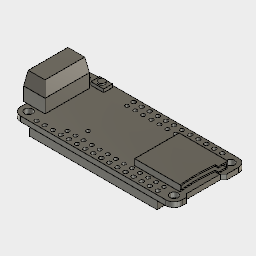
3436 Adafruit Music Maker Amp Feather Wing (Autodesk Fusion 360 design; units mm, degrees)
Autodesk Fusion 360 part; units mm, degrees
sketch "Adafruit VS1053 Amp FeatherWing" plane through (0, 0, 0) normal (0, 0, 1) x (1, 0, 0)
  line L0 (50.8, 16.637) -> (49.784, 15.621)
  line L1 (50.8, 3.937) -> (50.8, 2.54)
  line L2 (48.26, 0) -> (2.54, 0)
  line L3 (49.784, 15.621) -> (49.784, 4.953)
  line L4 (49.784, 4.953) -> (50.8, 3.937)
  line L5 (50.8, 20.32) -> (50.8, 16.637)
  circle A0 centre (48.26, 20.32) radius 1.27
  arc A1 (48.26, 0) -> (50.8, 2.54) centre (48.26, 2.54) ccw
  line L6 (2.54, 22.86) -> (48.26, 22.86)
  arc A2 (50.8, 20.32) -> (48.26, 22.86) centre (48.26, 20.32) ccw
  line L7 (0, 2.54) -> (0, 20.32)
  arc A3 (2.54, 22.86) -> (0, 20.32) centre (2.54, 20.32) ccw
  circle A4 centre (48.26, 2.54) radius 1.27
  arc A5 (0, 2.54) -> (2.54, 0) centre (2.54, 2.54) ccw
  circle A6 centre (13.97, 3.302) radius 0.8382
  circle A7 centre (16.51, 3.302) radius 0.8382
  circle A8 centre (19.05, 3.302) radius 0.8382
  circle A9 centre (39.37, 1.27) radius 0.889
  circle A10 centre (21.59, 3.302) radius 0.8382
  circle A11 centre (16.51, 3.302) radius 0.8382
  circle A12 centre (13.97, 3.302) radius 0.8382
  circle A13 centre (17.272, 6.5405) radius 0.8382
  circle A14 centre (19.05, 3.302) radius 0.8382
  circle A15 centre (2.159, 9.701) radius 1.0922
  circle A16 centre (29.21, 1.27) radius 0.889
  circle A17 centre (29.21, 1.27) radius 0.889
  circle A18 centre (44.45, 1.27) radius 0.889
  circle A19 centre (44.45, 1.27) radius 0.889
  circle A20 centre (26.67, 1.27) radius 0.889
  circle A21 centre (34.29, 21.59) radius 0.889
  circle A22 centre (34.29, 21.59) radius 0.889
  circle A23 centre (24.13, 3.302) radius 0.8382
  circle A24 centre (36.83, 21.59) radius 0.889
  circle A25 centre (36.83, 1.27) radius 0.889
  circle A26 centre (26.67, 1.27) radius 0.889
  circle A27 centre (24.13, 3.302) radius 0.8382
  circle A28 centre (19.05, 1.27) radius 0.889
  circle A29 centre (36.83, 21.59) radius 0.889
  circle A30 centre (6.35, 1.27) radius 0.889
  circle A31 centre (17.272, 6.5405) radius 0.8382
  circle A32 centre (21.59, 3.302) radius 0.8382
  circle A33 centre (8.89, 1.27) radius 0.889
  circle A34 centre (24.13, 1.27) radius 0.889
  circle A35 centre (26.67, 3.302) radius 0.8382
  circle A36 centre (26.67, 3.302) radius 0.8382
  circle A37 centre (29.21, 3.302) radius 0.8382
  circle A38 centre (8.89, 1.27) radius 0.889
  circle A39 centre (26.67, 21.59) radius 0.889
  circle A40 centre (6.35, 1.27) radius 0.889
  circle A41 centre (24.13, 21.59) radius 0.889
  circle A42 centre (11.43, 1.27) radius 0.889
  circle A43 centre (24.13, 21.59) radius 0.889
  circle A44 centre (21.59, 21.59) radius 0.889
  circle A45 centre (36.83, 1.27) radius 0.889
  circle A46 centre (39.37, 3.302) radius 0.8382
  circle A47 centre (34.29, 1.27) radius 0.889
  circle A48 centre (34.29, 1.27) radius 0.889
  circle A49 centre (24.13, 1.27) radius 0.889
  circle A50 centre (21.59, 1.27) radius 0.889
  circle A51 centre (21.59, 1.27) radius 0.889
  circle A52 centre (19.05, 1.27) radius 0.889
  circle A53 centre (39.37, 21.59) radius 0.889
  circle A54 centre (41.91, 21.59) radius 0.889
  circle A55 centre (39.37, 21.59) radius 0.889
  circle A56 centre (41.91, 21.59) radius 0.889
  circle A57 centre (31.75, 1.27) radius 0.889
  circle A58 centre (31.75, 1.27) radius 0.889
  circle A59 centre (41.91, 1.27) radius 0.889
  circle A60 centre (34.29, 3.302) radius 0.8382
  circle A61 centre (36.83, 3.302) radius 0.8382
  circle A62 centre (36.83, 3.302) radius 0.8382
  circle A63 centre (39.37, 1.27) radius 0.889
  circle A64 centre (44.45, 19.558) radius 0.8382
  circle A65 centre (39.37, 3.302) radius 0.8382
  circle A66 centre (41.91, 3.302) radius 0.8382
  circle A67 centre (41.91, 3.302) radius 0.8382
  circle A68 centre (44.45, 3.302) radius 0.8382
  circle A69 centre (44.45, 3.302) radius 0.8382
  circle A70 centre (44.45, 19.558) radius 0.8382
  circle A71 centre (41.91, 19.558) radius 0.8382
  circle A72 centre (39.37, 19.558) radius 0.8382
  circle A73 centre (41.91, 19.558) radius 0.8382
  circle A74 centre (39.37, 19.558) radius 0.8382
  circle A75 centre (31.75, 19.558) radius 0.8382
  circle A76 centre (36.83, 19.558) radius 0.8382
  circle A77 centre (29.21, 3.302) radius 0.8382
  circle A78 centre (31.75, 3.302) radius 0.8382
  circle A79 centre (31.75, 3.302) radius 0.8382
  circle A80 centre (34.29, 3.302) radius 0.8382
  circle A81 centre (36.83, 19.558) radius 0.8382
  circle A82 centre (34.29, 19.558) radius 0.8382
  circle A83 centre (34.29, 19.558) radius 0.8382
  circle A84 centre (26.67, 19.558) radius 0.8382
  circle A85 centre (31.75, 19.558) radius 0.8382
  circle A86 centre (29.21, 19.558) radius 0.8382
  circle A87 centre (29.21, 19.558) radius 0.8382
  circle A88 centre (26.67, 19.558) radius 0.8382
  circle A89 centre (19.05, 19.558) radius 0.8382
  circle A90 centre (24.13, 19.558) radius 0.8382
  circle A91 centre (24.13, 19.558) radius 0.8382
  circle A92 centre (21.59, 19.558) radius 0.8382
  circle A93 centre (21.59, 19.558) radius 0.8382
  circle A94 centre (2.159, 9.701) radius 1.0922
  circle A95 centre (19.05, 19.558) radius 0.8382
  circle A96 centre (16.51, 19.558) radius 0.8382
  circle A97 centre (16.51, 19.558) radius 0.8382
  circle A98 centre (2.159, 6.201) radius 1.0922
  circle A99 centre (2.159, 6.201) radius 1.0922
  circle A100 centre (2.159, 16.813) radius 1.0922
  circle A101 centre (2.159, 16.813) radius 1.0922
  circle A102 centre (2.159, 13.313) radius 1.0922
  circle A103 centre (2.159, 13.313) radius 1.0922
  circle A104 centre (41.91, 1.27) radius 0.889
  circle A105 centre (44.45, 21.59) radius 0.889
  circle A106 centre (16.51, 1.27) radius 0.889
  circle A107 centre (44.45, 21.59) radius 0.889
  circle A108 centre (31.75, 21.59) radius 0.889
  circle A109 centre (26.67, 21.59) radius 0.889
  circle A110 centre (16.51, 1.27) radius 0.889
  circle A111 centre (29.21, 21.59) radius 0.889
  circle A112 centre (13.97, 1.27) radius 0.889
  circle A113 centre (29.21, 21.59) radius 0.889
  circle A114 centre (13.97, 1.27) radius 0.889
  circle A115 centre (31.75, 21.59) radius 0.889
  circle A116 centre (11.43, 1.27) radius 0.889
  circle A117 centre (2.54, 20.32) radius 1.905
  circle A118 centre (21.59, 21.59) radius 0.889
  circle A119 centre (16.51, 21.59) radius 0.889
  circle A120 centre (16.51, 21.59) radius 0.889
  circle A121 centre (19.05, 21.59) radius 0.889
  circle A122 centre (2.54, 20.32) radius 1.905
  circle A123 centre (19.05, 21.59) radius 0.889
  circle A124 centre (2.54, 2.54) radius 1.905
  circle A125 centre (2.54, 2.54) radius 1.905
extrude "Extrude1" add sketch "Adafruit VS1053 Amp FeatherWing" along normal blind 1.6 makes body 1
move_face "OffsetFaces1" offset 0.635 2 faces at (4.4355, 20.1303, 1.0667) (4.4355, 2.3503, 1.0667) on bodies 1
move_face "OffsetFaces2" offset 0.254 58 faces at (17.0289, 22.3118, 0.5333) (18.1786, 21.4138, 1.0667) (20.7186, 21.4138, 1.0667) (22.4116, 19.7241, 0.5333) (19.8716, 19.7241, 0.5333) (17.3316, 19.7241, 0.5333) (23.2586, 21.4138, 1.0667) (24.9516, 19.7241, 0.5333) (25.7986, 21.4138, 1.0667) (27.4916, 19.7241, 0.5333) (28.3386, 21.4138, 1.0667) (30.0316, 19.7241, 0.5333) (32.1556, 22.3811, 0.5333) (32.2048, 18.8539, 0.5333) (34.3122, 22.4787, 1.0667) (33.6479, 19.0192, 1.0667) (36.8522, 22.4787, 1.0667) (36.1879, 19.0192, 1.0667) (39.3922, 22.4787, 1.0667) (38.7279, 19.0192, 1.0667) (41.9322, 22.4787, 1.0667) (41.2679, 19.0192, 1.0667) (44.4722, 22.4787, 1.0667) (43.8079, 19.0192, 1.0667) (18.1092, 6.5823, 0.5333) (14.8072, 3.3438, 0.5333) (14.8579, 1.3143, 0.5333) (12.3179, 1.3143, 0.5333) (9.7779, 1.3143, 0.5333) (7.2379, 1.3143, 0.5333) (16.7508, 0.4142, 0.5333) (17.3472, 3.3438, 0.5333) (19.8872, 3.3438, 0.5333) (19.2908, 0.4142, 0.5333) (22.4272, 3.3438, 0.5333) (21.8308, 0.4142, 0.5333) (24.9672, 3.3438, 0.5333) (24.3708, 0.4142, 0.5333) (26.9108, 0.4142, 0.5333) (27.5072, 3.3438, 0.5333) (30.0472, 3.3438, 0.5333) (29.4508, 0.4142, 0.5333) (32.1556, 2.0611, 0.5333) (32.2048, 2.5979, 0.5333) (34.4356, 4.1275, 0.5333) (34.3122, 2.1587, 1.0667) (36.8522, 2.1587, 1.0667) (36.9756, 4.1275, 0.5333) (39.5156, 4.1275, 0.5333) (39.3922, 2.1587, 1.0667) (41.9322, 2.1587, 1.0667) (42.0556, 4.1275, 0.5333) (44.5956, 4.1275, 0.5333) (44.4722, 2.1587, 1.0667) (3.2498, 6.2554, 0.5333) (3.2498, 9.7554, 0.5333) (3.2498, 13.3674, 0.5333) (3.2498, 16.8674, 0.5333) on bodies 1
sketch "terminal" plane through (0, 0, 1.6) normal (0, 0, 1) x (-1, 0, 0)
  circle A0 centre (-17.272, -6.5405) radius 0.5842
  circle A1 centre (-44.45, -1.27) radius 0.635
  circle A2 centre (-24.13, -3.302) radius 0.5842
  circle A3 centre (-34.29, -21.59) radius 0.635
  circle A4 centre (-26.67, -1.27) radius 0.635
  circle A5 centre (-29.21, -1.27) radius 0.635
  circle A6 centre (-41.91, -21.59) radius 0.635
  circle A7 centre (-26.67, -21.59) radius 0.635
  circle A8 centre (-41.91, -1.27) radius 0.635
  circle A9 centre (-34.29, -1.27) radius 0.635
  circle A10 centre (-6.35, -1.27) radius 0.635
  circle A11 centre (-44.45, -21.59) radius 0.635
  circle A12 centre (-21.59, -3.302) radius 0.5842
  circle A13 centre (-2.159, -6.201) radius 0.8382
  circle A14 centre (-39.37, -21.59) radius 0.635
  circle A15 centre (-24.13, -21.59) radius 0.635
  circle A16 centre (-26.67, -3.302) radius 0.5842
  circle A17 centre (-21.59, -1.27) radius 0.635
  circle A18 centre (-8.89, -1.27) radius 0.635
  circle A19 centre (-19.05, -1.27) radius 0.635
  circle A20 centre (-48.26, -20.32) radius 1.27
  circle A21 centre (-16.51, -1.27) radius 0.635
  circle A22 centre (-29.21, -21.59) radius 0.635
  circle A23 centre (-13.97, -1.27) radius 0.635
  circle A24 centre (-31.75, -21.59) radius 0.635
  circle A25 centre (-11.43, -1.27) radius 0.635
  circle A26 centre (-21.59, -21.59) radius 0.635
  circle A27 centre (-16.51, -21.59) radius 0.635
  circle A28 centre (-2.54, -20.32) radius 1.27
  circle A29 centre (-19.05, -21.59) radius 0.635
  circle A30 centre (-2.54, -2.54) radius 1.27
  circle A31 centre (-16.51, -19.558) radius 0.5842
  circle A32 centre (-19.05, -19.558) radius 0.5842
  circle A33 centre (-36.83, -21.59) radius 0.635
  circle A34 centre (-24.13, -1.27) radius 0.635
  circle A35 centre (-2.159, -16.813) radius 0.8382
  circle A36 centre (-36.83, -1.27) radius 0.635
  circle A37 centre (-2.159, -13.313) radius 0.8382
  circle A38 centre (-16.51, -3.302) radius 0.5842
  circle A39 centre (-26.67, -19.558) radius 0.5842
  circle A40 centre (-13.97, -3.302) radius 0.5842
  circle A41 centre (-19.05, -3.302) radius 0.5842
  circle A42 centre (-21.59, -19.558) radius 0.5842
  circle A43 centre (-24.13, -19.558) radius 0.5842
  circle A44 centre (-31.75, -19.558) radius 0.5842
  circle A45 centre (-34.29, -19.558) radius 0.5842
  circle A46 centre (-36.83, -19.558) radius 0.5842
  circle A47 centre (-34.29, -3.302) radius 0.5842
  circle A48 centre (-31.75, -3.302) radius 0.5842
  circle A49 centre (-29.21, -3.302) radius 0.5842
  circle A50 centre (-39.37, -19.558) radius 0.5842
  circle A51 centre (-41.91, -19.558) radius 0.5842
  circle A52 centre (-44.45, -19.558) radius 0.5842
  circle A53 centre (-44.45, -3.302) radius 0.5842
  circle A54 centre (-41.91, -3.302) radius 0.5842
  circle A55 centre (-39.37, -3.302) radius 0.5842
  circle A56 centre (-39.37, -1.27) radius 0.635
  circle A57 centre (-36.83, -3.302) radius 0.5842
  circle A58 centre (-31.75, -1.27) radius 0.635
  circle A59 centre (-48.26, -2.54) radius 1.27
  circle A60 centre (-29.21, -19.558) radius 0.5842
  circle A61 centre (-2.159, -9.701) radius 0.8382
  arc A62 (-2.54, -22.86) -> (0, -20.32) centre (-2.54, -20.32) ccw
  line L0 (0, -20.32) -> (0, -2.54)
  arc A63 (0, -2.54) -> (-2.54, 0) centre (-2.54, -2.54) ccw
  line L1 (-2.54, 0) -> (-48.26, 0)
  arc A64 (-48.26, 0) -> (-50.8, -2.54) centre (-48.26, -2.54) ccw
  line L2 (-50.8, -2.54) -> (-50.8, -3.937)
  line L3 (-50.8, -3.937) -> (-49.784, -4.953)
  line L4 (-49.784, -4.953) -> (-49.784, -15.621)
  line L5 (-49.784, -15.621) -> (-50.8, -16.637)
  line L6 (-50.8, -16.637) -> (-50.8, -20.32)
  arc A65 (-50.8, -20.32) -> (-48.26, -22.86) centre (-48.26, -20.32) ccw
  line L7 (-48.26, -22.86) -> (-2.54, -22.86)
  line L8 (1, -18.43) -> (-5.8, -18.43)
  line L9 (-5.8, -18.43) -> (-5.8, -4.43)
  line L10 (-5.8, -4.43) -> (1, -4.43)
  line L11 (1, -4.43) -> (1, -18.43)
  line L12 (-5.8, -11.43) -> (1, -11.43) construction
  line L13 (0, -11.43) -> (-58, -11.43) construction
  dimension "d5" = 14
  dimension "d6" = 6.8
  dimension "d7" = 1
  measures "d5" distance of L8.start L10.end
  measures "d6" distance of L8.start L8.end
  measures "d7" distance of L0 L11
extrude "Extrude2" add sketch "terminal" along normal blind 4.25 separate body contours A13 | A35 | A37 | A61 | L0 L8 L9 L10 | L0 L8 L10 L11 makes body 2
sketch "terminal 2" plane through (0, 0, 5.85) normal (0, 0, 1) x (-1, 0, 0)
  line L0 (1, -4.43) -> (-5.8, -4.43)
  line L1 (-5.8, -4.43) -> (-5.8, -18.43)
  line L2 (-5.8, -18.43) -> (1, -18.43)
  line L3 (1, -18.43) -> (1, -4.43)
extrude "Extrude3" add sketch "terminal 2" along normal blind 4.25 draft -10 bodies 2
sketch "RESET" plane through (0, 0, 1.6) normal (0, 0, 1) x (-1, 0, 0)
  circle A0 centre (-17.272, -6.5405) radius 0.5842
  circle A1 centre (-44.45, -1.27) radius 0.635
  circle A2 centre (-24.13, -3.302) radius 0.5842
  circle A3 centre (-34.29, -21.59) radius 0.635
  circle A4 centre (-26.67, -1.27) radius 0.635
  circle A5 centre (-29.21, -1.27) radius 0.635
  circle A6 centre (-41.91, -21.59) radius 0.635
  circle A7 centre (-26.67, -21.59) radius 0.635
  circle A8 centre (-41.91, -1.27) radius 0.635
  circle A9 centre (-34.29, -1.27) radius 0.635
  circle A10 centre (-6.35, -1.27) radius 0.635
  circle A11 centre (-44.45, -21.59) radius 0.635
  circle A12 centre (-21.59, -3.302) radius 0.5842
  circle A13 centre (-2.159, -6.201) radius 0.8382
  circle A14 centre (-39.37, -21.59) radius 0.635
  circle A15 centre (-24.13, -21.59) radius 0.635
  circle A16 centre (-26.67, -3.302) radius 0.5842
  circle A17 centre (-21.59, -1.27) radius 0.635
  circle A18 centre (-8.89, -1.27) radius 0.635
  circle A19 centre (-19.05, -1.27) radius 0.635
  circle A20 centre (-48.26, -20.32) radius 1.27
  circle A21 centre (-16.51, -1.27) radius 0.635
  circle A22 centre (-29.21, -21.59) radius 0.635
  circle A23 centre (-13.97, -1.27) radius 0.635
  circle A24 centre (-31.75, -21.59) radius 0.635
  circle A25 centre (-11.43, -1.27) radius 0.635
  circle A26 centre (-21.59, -21.59) radius 0.635
  circle A27 centre (-16.51, -21.59) radius 0.635
  circle A28 centre (-2.54, -20.32) radius 1.27
  circle A29 centre (-19.05, -21.59) radius 0.635
  circle A30 centre (-2.54, -2.54) radius 1.27
  circle A31 centre (-16.51, -19.558) radius 0.5842
  circle A32 centre (-19.05, -19.558) radius 0.5842
  circle A33 centre (-36.83, -21.59) radius 0.635
  circle A34 centre (-24.13, -1.27) radius 0.635
  circle A35 centre (-2.159, -16.813) radius 0.8382
  circle A36 centre (-36.83, -1.27) radius 0.635
  circle A37 centre (-2.159, -13.313) radius 0.8382
  circle A38 centre (-16.51, -3.302) radius 0.5842
  circle A39 centre (-26.67, -19.558) radius 0.5842
  circle A40 centre (-13.97, -3.302) radius 0.5842
  circle A41 centre (-19.05, -3.302) radius 0.5842
  circle A42 centre (-21.59, -19.558) radius 0.5842
  circle A43 centre (-24.13, -19.558) radius 0.5842
  circle A44 centre (-31.75, -19.558) radius 0.5842
  circle A45 centre (-34.29, -19.558) radius 0.5842
  circle A46 centre (-36.83, -19.558) radius 0.5842
  circle A47 centre (-34.29, -3.302) radius 0.5842
  circle A48 centre (-31.75, -3.302) radius 0.5842
  circle A49 centre (-29.21, -3.302) radius 0.5842
  circle A50 centre (-39.37, -19.558) radius 0.5842
  circle A51 centre (-41.91, -19.558) radius 0.5842
  circle A52 centre (-44.45, -19.558) radius 0.5842
  circle A53 centre (-44.45, -3.302) radius 0.5842
  circle A54 centre (-41.91, -3.302) radius 0.5842
  circle A55 centre (-39.37, -3.302) radius 0.5842
  circle A56 centre (-39.37, -1.27) radius 0.635
  circle A57 centre (-36.83, -3.302) radius 0.5842
  circle A58 centre (-31.75, -1.27) radius 0.635
  circle A59 centre (-48.26, -2.54) radius 1.27
  circle A60 centre (-29.21, -19.558) radius 0.5842
  circle A61 centre (-2.159, -9.701) radius 0.8382
  arc A62 (-2.54, -22.86) -> (0, -20.32) centre (-2.54, -20.32) ccw
  line L0 (0, -20.32) -> (0, -2.54)
  arc A63 (0, -2.54) -> (-2.54, 0) centre (-2.54, -2.54) ccw
  line L1 (-2.54, 0) -> (-48.26, 0)
  arc A64 (-48.26, 0) -> (-50.8, -2.54) centre (-48.26, -2.54) ccw
  line L2 (-50.8, -2.54) -> (-50.8, -3.937)
  line L3 (-50.8, -3.937) -> (-49.784, -4.953)
  line L4 (-49.784, -4.953) -> (-49.784, -15.621)
  line L5 (-49.784, -15.621) -> (-50.8, -16.637)
  line L6 (-50.8, -16.637) -> (-50.8, -20.32)
  arc A65 (-50.8, -20.32) -> (-48.26, -22.86) centre (-48.26, -20.32) ccw
  line L7 (-48.26, -22.86) -> (-2.54, -22.86)
  line L8 (-5.239, -22.228) -> (-9.239, -22.228)
  line L9 (-9.239, -22.228) -> (-9.239, -19.428)
  line L10 (-9.239, -19.428) -> (-5.239, -19.428)
  line L11 (-5.239, -19.428) -> (-5.239, -22.228)
  line L12 (-7.239, -22.228) -> (-7.239, -19.428) construction
  line L13 (-9.239, -20.828) -> (-5.239, -20.828) construction
  circle A66 centre (-7.239, -20.828) radius 1
  dimension "d12" = 4
  dimension "d13" = 2.8
  dimension "d14" = 2
  dimension "d15" = 7.239
  dimension "d16" = 20.828
  measures "d12" distance of L8.start L8.end
  measures "d13" distance of L8.start L10.end
  measures "d14" diameter of A66
  measures "d15" distance of L0 L12
  measures "d16" distance of L1 L13
extrude "Extrude4" add sketch "RESET" along normal blind 1 separate body contours L8 L9 L10 L11 | A66 makes body 3
extrude "Extrude5" add sketch "RESET" along normal blind 0.5 from surface at 1 contours A66 bodies 3
sketch "sd card" plane through (0, 0, 1.6) normal (0, 0, 1) x (-1, 0, 0)
  circle A0 centre (-17.272, -6.5405) radius 0.5842
  circle A1 centre (-44.45, -1.27) radius 0.635
  circle A2 centre (-24.13, -3.302) radius 0.5842
  circle A3 centre (-34.29, -21.59) radius 0.635
  circle A4 centre (-26.67, -1.27) radius 0.635
  circle A5 centre (-29.21, -1.27) radius 0.635
  circle A6 centre (-41.91, -21.59) radius 0.635
  circle A7 centre (-26.67, -21.59) radius 0.635
  circle A8 centre (-41.91, -1.27) radius 0.635
  circle A9 centre (-34.29, -1.27) radius 0.635
  circle A10 centre (-6.35, -1.27) radius 0.635
  circle A11 centre (-44.45, -21.59) radius 0.635
  circle A12 centre (-21.59, -3.302) radius 0.5842
  circle A13 centre (-2.159, -6.201) radius 0.8382
  circle A14 centre (-39.37, -21.59) radius 0.635
  circle A15 centre (-24.13, -21.59) radius 0.635
  circle A16 centre (-26.67, -3.302) radius 0.5842
  circle A17 centre (-21.59, -1.27) radius 0.635
  circle A18 centre (-8.89, -1.27) radius 0.635
  circle A19 centre (-19.05, -1.27) radius 0.635
  circle A20 centre (-48.26, -20.32) radius 1.27
  circle A21 centre (-16.51, -1.27) radius 0.635
  circle A22 centre (-29.21, -21.59) radius 0.635
  circle A23 centre (-13.97, -1.27) radius 0.635
  circle A24 centre (-31.75, -21.59) radius 0.635
  circle A25 centre (-11.43, -1.27) radius 0.635
  circle A26 centre (-21.59, -21.59) radius 0.635
  circle A27 centre (-16.51, -21.59) radius 0.635
  circle A28 centre (-2.54, -20.32) radius 1.27
  circle A29 centre (-19.05, -21.59) radius 0.635
  circle A30 centre (-2.54, -2.54) radius 1.27
  circle A31 centre (-16.51, -19.558) radius 0.5842
  circle A32 centre (-19.05, -19.558) radius 0.5842
  circle A33 centre (-36.83, -21.59) radius 0.635
  circle A34 centre (-24.13, -1.27) radius 0.635
  circle A35 centre (-2.159, -16.813) radius 0.8382
  circle A36 centre (-36.83, -1.27) radius 0.635
  circle A37 centre (-2.159, -13.313) radius 0.8382
  circle A38 centre (-16.51, -3.302) radius 0.5842
  circle A39 centre (-26.67, -19.558) radius 0.5842
  circle A40 centre (-13.97, -3.302) radius 0.5842
  circle A41 centre (-19.05, -3.302) radius 0.5842
  circle A42 centre (-21.59, -19.558) radius 0.5842
  circle A43 centre (-24.13, -19.558) radius 0.5842
  circle A44 centre (-31.75, -19.558) radius 0.5842
  circle A45 centre (-34.29, -19.558) radius 0.5842
  circle A46 centre (-36.83, -19.558) radius 0.5842
  circle A47 centre (-34.29, -3.302) radius 0.5842
  circle A48 centre (-31.75, -3.302) radius 0.5842
  circle A49 centre (-29.21, -3.302) radius 0.5842
  circle A50 centre (-39.37, -19.558) radius 0.5842
  circle A51 centre (-41.91, -19.558) radius 0.5842
  circle A52 centre (-44.45, -19.558) radius 0.5842
  circle A53 centre (-44.45, -3.302) radius 0.5842
  circle A54 centre (-41.91, -3.302) radius 0.5842
  circle A55 centre (-39.37, -3.302) radius 0.5842
  circle A56 centre (-39.37, -1.27) radius 0.635
  circle A57 centre (-36.83, -3.302) radius 0.5842
  circle A58 centre (-31.75, -1.27) radius 0.635
  circle A59 centre (-48.26, -2.54) radius 1.27
  circle A60 centre (-29.21, -19.558) radius 0.5842
  circle A61 centre (-2.159, -9.701) radius 0.8382
  arc A62 (-2.54, -22.86) -> (0, -20.32) centre (-2.54, -20.32) ccw
  line L0 (0, -20.32) -> (0, -2.54)
  arc A63 (0, -2.54) -> (-2.54, 0) centre (-2.54, -2.54) ccw
  line L1 (-2.54, 0) -> (-48.26, 0)
  arc A64 (-48.26, 0) -> (-50.8, -2.54) centre (-48.26, -2.54) ccw
  line L2 (-50.8, -2.54) -> (-50.8, -3.937)
  line L3 (-50.8, -3.937) -> (-49.784, -4.953)
  line L4 (-49.784, -4.953) -> (-49.784, -15.621)
  line L5 (-49.784, -15.621) -> (-50.8, -16.637)
  line L6 (-50.8, -16.637) -> (-50.8, -20.32)
  arc A65 (-50.8, -20.32) -> (-48.26, -22.86) centre (-48.26, -20.32) ccw
  line L7 (-48.26, -22.86) -> (-2.54, -22.86)
  line L8 (-34, -18.43) -> (-49.3, -18.43)
  line L9 (-49.3, -18.43) -> (-49.3, -4.43)
  line L10 (-49.3, -4.43) -> (-34, -4.43)
  line L11 (-34, -4.43) -> (-34, -18.43)
  line L12 (-34, -11.43) -> (-49.3, -11.43) construction
  line L13 (0, -11.43) -> (-28, -11.43) construction
  spline S0 degree 2 poles (-49, -20) (-47, -10) (-49, 0) knots 0 0 0 2.009975 2.009975 2.009975
  line L14 (-34, -15.43) -> (-49.3, -15.43)
  dimension "d22" = 15.3
  dimension "d23" = 14
  dimension "d24" = 1.5
  dimension "d26" = 3
  measures "d22" distance of L8.start L8.end
  measures "d23" distance of L8.start L10.end
  measures "d24" distance of L6 L9
  measures "d26" distance of L8 L14
extrude "Extrude6" add sketch "sd card" along normal blind 1.9 separate body contours L8 L11 S0 L14 | L8 L9 S0 L14 | L10 L11 S0 L14 makes body 4
shell "Shell1" thickness 0.4 removed faces 3 at (48.1444, 13.8004, 2.2333) at (49.3, 17.43, 2.2333) at (48.6299, 15.43, 2.2333) on bodies 4
sketch "terminal holes" plane through (-1, 0, 0) normal (-1, 0, 0) x (0, -1, 0)
  line L0 (-18.43, 1.6) -> (-4.43, 1.6)
  line L1 (-4.43, 1.6) -> (-4.43, 5.85)
  line L2 (-4.43, 5.85) -> (-18.43, 5.85)
  line L3 (-18.43, 5.85) -> (-18.43, 1.6)
  line L4 (-18.43, 3.5) -> (-4.43, 3.5) construction
  circle A0 centre (-16.68, 3.5) radius 1
  circle A1 centre (-13.18, 3.5) radius 1
  circle A2 centre (-9.68, 3.5) radius 1
  circle A3 centre (-6.18, 3.5) radius 1
  point P0 (-18.43, 3.5)
  point P1 (-4.43, 3.5)
  dimension "d30" = 2
  dimension "d31" = 1.75
  dimension "d34" = 3.5
  dimension "d35" = 0
  measures "d30" diameter of A0
  measures "d31" distance of L3 A0.centre
extrude "Extrude7" cut sketch "terminal holes" against normal blind 0.5 contours A0 | A1 | A2 | A3 bodies 2
sketch "headers" plane through (0, 0, 0) normal (0, 0, -1) x (1, 0, 0)
  circle A0 centre (17.272, -6.5405) radius 0.5842
  circle A1 centre (44.45, -1.27) radius 0.635
  circle A2 centre (24.13, -3.302) radius 0.5842
  circle A3 centre (34.29, -21.59) radius 0.635
  circle A4 centre (26.67, -1.27) radius 0.635
  circle A5 centre (29.21, -1.27) radius 0.635
  circle A6 centre (41.91, -21.59) radius 0.635
  circle A7 centre (26.67, -21.59) radius 0.635
  circle A8 centre (41.91, -1.27) radius 0.635
  circle A9 centre (34.29, -1.27) radius 0.635
  circle A10 centre (6.35, -1.27) radius 0.635
  circle A11 centre (44.45, -21.59) radius 0.635
  circle A12 centre (21.59, -3.302) radius 0.5842
  circle A13 centre (2.159, -6.201) radius 0.8382
  circle A14 centre (39.37, -21.59) radius 0.635
  circle A15 centre (24.13, -21.59) radius 0.635
  circle A16 centre (26.67, -3.302) radius 0.5842
  circle A17 centre (21.59, -1.27) radius 0.635
  circle A18 centre (8.89, -1.27) radius 0.635
  circle A19 centre (19.05, -1.27) radius 0.635
  circle A20 centre (48.26, -20.32) radius 1.27
  circle A21 centre (16.51, -1.27) radius 0.635
  circle A22 centre (29.21, -21.59) radius 0.635
  circle A23 centre (13.97, -1.27) radius 0.635
  circle A24 centre (31.75, -21.59) radius 0.635
  circle A25 centre (11.43, -1.27) radius 0.635
  circle A26 centre (21.59, -21.59) radius 0.635
  circle A27 centre (16.51, -21.59) radius 0.635
  circle A28 centre (2.54, -20.32) radius 1.27
  circle A29 centre (19.05, -21.59) radius 0.635
  circle A30 centre (2.54, -2.54) radius 1.27
  circle A31 centre (16.51, -19.558) radius 0.5842
  circle A32 centre (19.05, -19.558) radius 0.5842
  circle A33 centre (36.83, -21.59) radius 0.635
  circle A34 centre (24.13, -1.27) radius 0.635
  circle A35 centre (2.159, -16.813) radius 0.8382
  circle A36 centre (36.83, -1.27) radius 0.635
  circle A37 centre (2.159, -13.313) radius 0.8382
  circle A38 centre (16.51, -3.302) radius 0.5842
  circle A39 centre (26.67, -19.558) radius 0.5842
  circle A40 centre (13.97, -3.302) radius 0.5842
  circle A41 centre (19.05, -3.302) radius 0.5842
  circle A42 centre (21.59, -19.558) radius 0.5842
  circle A43 centre (24.13, -19.558) radius 0.5842
  circle A44 centre (31.75, -19.558) radius 0.5842
  circle A45 centre (34.29, -19.558) radius 0.5842
  circle A46 centre (36.83, -19.558) radius 0.5842
  circle A47 centre (34.29, -3.302) radius 0.5842
  circle A48 centre (31.75, -3.302) radius 0.5842
  circle A49 centre (29.21, -3.302) radius 0.5842
  circle A50 centre (39.37, -19.558) radius 0.5842
  circle A51 centre (41.91, -19.558) radius 0.5842
  circle A52 centre (44.45, -19.558) radius 0.5842
  circle A53 centre (44.45, -3.302) radius 0.5842
  circle A54 centre (41.91, -3.302) radius 0.5842
  circle A55 centre (39.37, -3.302) radius 0.5842
  circle A56 centre (39.37, -1.27) radius 0.635
  circle A57 centre (36.83, -3.302) radius 0.5842
  circle A58 centre (31.75, -1.27) radius 0.635
  circle A59 centre (48.26, -2.54) radius 1.27
  circle A60 centre (29.21, -19.558) radius 0.5842
  circle A61 centre (2.159, -9.701) radius 0.8382
  arc A62 (0, -20.32) -> (2.54, -22.86) centre (2.54, -20.32) ccw
  line L0 (2.54, -22.86) -> (48.26, -22.86)
  arc A63 (48.26, -22.86) -> (50.8, -20.32) centre (48.26, -20.32) ccw
  line L1 (50.8, -20.32) -> (50.8, -16.637)
  line L2 (50.8, -16.637) -> (49.784, -15.621)
  line L3 (49.784, -15.621) -> (49.784, -4.953)
  line L4 (49.784, -4.953) -> (50.8, -3.937)
  line L5 (50.8, -3.937) -> (50.8, -2.54)
  arc A64 (50.8, -2.54) -> (48.26, 0) centre (48.26, -2.54) ccw
  line L6 (48.26, 0) -> (2.54, 0)
  arc A65 (2.54, 0) -> (0, -2.54) centre (2.54, -2.54) ccw
  line L7 (0, -2.54) -> (0, -20.32)
  line L8 (5.35, 0) -> (45.45, 0)
  line L9 (45.45, 0) -> (45.45, -2.5)
  line L10 (45.45, -2.5) -> (5.35, -2.5)
  line L11 (5.35, -2.5) -> (5.35, 0)
  line L12 (45.45, -22.86) -> (15.51, -22.86)
  line L13 (15.51, -22.86) -> (15.51, -20.36)
  line L14 (15.51, -20.36) -> (45.45, -20.36)
  line L15 (45.45, -20.36) -> (45.45, -22.86)
  dimension "d38" = 2.5
  dimension "d39" = 1
  dimension "d40" = 1
  dimension "d43" = 2.5
  dimension "d44" = 1
  dimension "d45" = 1
  measures "d38" distance of L8.end L9.end
  measures "d39" distance of A1.centre L9
  measures "d40" distance of A10.centre L11
  measures "d43" distance of L12.end L13.end
  measures "d44" distance of A27.centre L13
  measures "d45" distance of A11.centre L15
extrude "Extrude8" add sketch "headers" along normal blind 2.5 separate body contours A1 | A3 | A4 | A5 | A6 | A7 | A8 | A9 | A10 | A11 | A14 | A15 | A17 | A18 | A19 | A21 | A22 | A23 | A24 | A25 | A26 | A27 | A29 | A33 | A34 | A36 | A56 | A58 | L0 L12 L13 L14 L15 | L6 L8 L9 L10 L11 makes body 5 at (18.7167, 0.8333, 0) makes body 6 at (25.49, 21.1933, 0)
equation "d3 = ( 1.27 / 2 ) * 1 mm"
equation "d4 = ( 0.508 / 2 ) * 1 mm"
equation "d8 = ( 8.500 / 2 ) * 1 mm"
equation "d10 = ( 8.5 / 2 ) * 1 mm"
equation "d31 = ( 3.5 / 2 ) * 1 mm"
named bodies: "PCB", "terminal audio", "reset", "sd holder"
